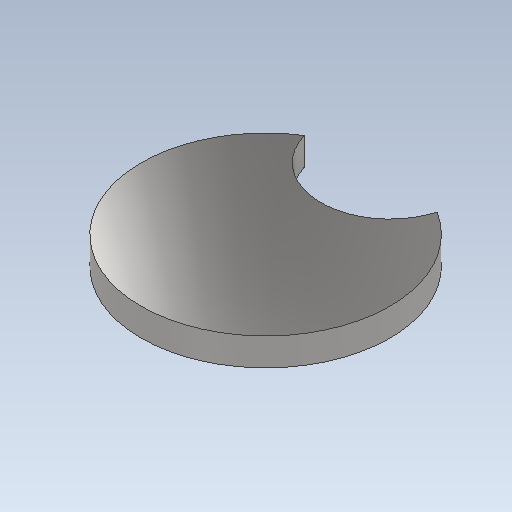
# Autodesk Inventor part: Pieza6
Saved by Autodesk Inventor 2020.3 (Build 243373000, 373)
## iProperties
Created: 2020-12-07
Part Number: Pieza6
Material: Acero inoxidable
Document SubType Name: Modeling
Designer: codig
Density: 8 g/cm^3
Appearance: Semipulido
Author: codig
Autodesk Inventor part; units mm, degrees
ref_plane "YZ Plane" through (0, 0, 0) normal (1, 0, 0) x (0, 1, 0)
ref_plane "XZ Plane" through (0, 0, 0) normal (0, 1, 0) x (-1, 0, 0)
ref_plane "XY Plane" through (0, 0, 0) normal (0, 0, 1) x (1, 0, 0)
sketch "Boceto1" plane through (0, 0, 0) normal (0, 1, 0) x (-1, 0, 0)
  arc A0 (12.0081, -19.0278) -> (-12.0081, -19.0278) centre (0, 0) ccw
  arc A1 (12.0081, -19.0278) -> (-12.0081, -19.0278) centre (0, -22.5) ccw
  constraints: 4 point on circle, 2 centre point
extrude "Extrusión1" add sketch "Boceto1" along normal blind 5
